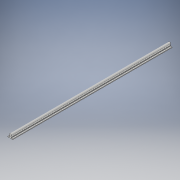
# Autodesk Inventor part: 1000mmFührung
Saved by Autodesk Inventor 2019 (Build 230136000, 136)
## iProperties
Created: 2021-05-01
Part Number: 1000mmFührung
Material: Generic
Document SubType Name: Modeling
Designer: Michael Sumper
Density: 1 g/cm^3
Appearance: Default
Author: Michael Sumper
Autodesk Inventor part; units mm, degrees
ref_plane "YZ Plane" through (0, 0, 0) normal (1, 0, 0) x (0, 1, 0)
ref_plane "XZ Plane" through (0, 0, 0) normal (0, 1, 0) x (-1, 0, 0)
ref_plane "XY Plane" through (0, 0, 0) normal (0, 0, 1) x (1, 0, 0)
sketch "Skizze1" plane through (0, 0, 0) normal (0, 0, 1) x (1, 0, 0)
  line L0 (-15, 2) -> (-15, -2)
  line L1 (-15, -2) -> (15, -2)
  line L2 (15, -2) -> (15, 2)
  line L3 (15, 2) -> (-15, -2) construction
  line L4 (-15, 2) -> (15, -2) construction
  line L5 (-15, 2) -> (-6.65, 2) construction
  line L6 (15, 2) -> (6.65, 2) construction
  line L7 (-6.65, 2) -> (-6.65, 6)
  line L8 (-6.65, 6) -> (-5.387, 6)
  line L9 (6.65, 2) -> (6.65, 6)
  line L10 (6.65, 6) -> (5.387, 6)
  line L11 (-5.387, 6) -> (-2.248, 11.4369)
  line L12 (-5.387, 6) -> (0.891, 6) construction
  line L13 (5.387, 6) -> (2.248, 11.4369)
  line L14 (5.387, 6) -> (11.665, 6) construction
  arc A0 (2.248, 11.4369) -> (-2.248, 11.4369) centre (0, 16.9999) ccw
  line L15 (15, 2) -> (6.65, 2)
  line L16 (-6.65, 2) -> (-15, 2)
  point P0 (0, 0)
  dimension "d0" = 30
  dimension "d1" = 4
  dimension "d2" = 8.35
  dimension "d3" = 8.35
  dimension "d4" = 4
  dimension "d5" = 1.263
  dimension "d6" = 4
  dimension "d7" = 1.263
  dimension "d8" = 6.278
  dimension "d9" = 60
  dimension "d10" = 6.278
  dimension "d11" = 120
  dimension "d12" = 6
  constraints: 34 end point, 6 horizontal, 3 parallel, 3 perpendicular, 2 equal length, 2 midpoint, 2 point on circle, 2 vertical, 1 centre point
  measures "d0" distance of L1.end L0.end
  measures "d1" distance of L0.end L0.start
  measures "d2" distance of L0.start L5.end
  measures "d3" distance of L2.end L6.end
  measures "d4" distance of L5.end L7.end
  measures "d5" distance of L7.end L8.end
  measures "d6" distance of L6.end L9.end
  measures "d7" distance of L9.end L10.end
  measures "d8" distance of L8.end L11.end
  measures "d9" angle of L12 L11
  measures "d10" distance of L10.end L13.end
  measures "d11" angle of L14 L13
  measures "d12" radius of A0
extrude "Extrusion1" add sketch "Skizze1" along normal blind 1000
